Autodesk Inventor part; units mm, degrees
(part 14 of 16)
  arc A294 (20.5053, 59.1049) -> (19.7702, 59.9479) centre (0.0409, 42.0024) ccw
  spline S90 degree 3 poles (17.578, 62.0957) (17.5149, 61.9054) (17.4259, 61.6609) (17.3048, 61.369) (17.2372, 61.2153) (17.171, 61.0728) (17.1066, 60.9415) (17.0444, 60.8212) (16.9848, 60.7117) (16.9284, 60.6129) (16.8755, 60.5246) (16.8265, 60.4466) (16.7818, 60.3788) (16.7419, 60.3207) (16.7071, 60.2724) (16.6673, 60.2192) (16.6296, 60.1737) (16.5954, 60.1304) (16.5731, 60.101) (16.5518, 60.0719) (16.5315, 60.0431) (16.5122, 60.0145) (16.494, 59.9861) (16.4767, 59.9579) (16.4604, 59.9297) (16.4451, 59.9016) (16.4307, 59.8733) (16.4173, 59.8448) (16.4048, 59.8159) (16.3933, 59.7865) (16.3828, 59.7562) (16.3735, 59.7248) (16.3654, 59.6921) (16.3588, 59.6574) (16.354, 59.6205) (16.3517, 59.5807) (16.3525, 59.5377) (16.3576, 59.4911) (16.3684, 59.4408) (16.3865, 59.3878) (16.4133, 59.3335) (16.4479, 59.2826) (16.5472, 59.1764) (16.7178, 59.0249) (16.8727, 58.8575) (16.981, 58.7604) (17.0325, 58.7268) (17.0873, 58.7011) (17.1408, 58.6842) (17.1912, 58.6744) (17.2379, 58.6703) (17.281, 58.6703) (17.3207, 58.6735) (17.3575, 58.679) (17.392, 58.6863) (17.4246, 58.695) (17.4558, 58.705) (17.4858, 58.7161) (17.515, 58.7283) (17.5436, 58.7413) (17.5718, 58.7554) (17.5998, 58.7703) (17.6277, 58.7862) (17.6555, 58.8031) (17.6834, 58.8209) (17.7114, 58.8398) (17.7396, 58.8596) (17.7679, 58.8804) (17.7966, 58.9023) (17.8255, 58.9253) (17.8681, 58.9603) (17.9128, 58.999) (17.9652, 59.0398) (18.0128, 59.0757) (18.07, 59.1168) (18.137, 59.1628) (18.2139, 59.2134) (18.3011, 59.2681) (18.3987, 59.3265) (18.5069, 59.3883) (18.626, 59.453) (18.7559, 59.5201) (18.897, 59.5892) (19.0493, 59.66) (19.3387, 59.787) (19.5813, 59.881) (19.7702, 59.9479) knots 0 0 0 0 0.085622 0.111078 0.134991 0.157361 0.178189 0.197474 0.215216 0.231415 0.246072 0.259186 0.270757 0.280785 0.28927 0.296213 0.309142 0.314525 0.319779 0.32491 0.329923 0.334826 0.339627 0.344336 0.348964 0.353525 0.358035 0.362514 0.366985 0.371475 0.37602 0.380661 0.385447 0.39044 0.395711 0.401345 0.407436 0.41408 0.421363 0.429333 0.437971 0.447155 0.455484 0.5 0.544516 0.552845 0.562029 0.570667 0.578637 0.58592 0.592564 0.598655 0.604289 0.60956 0.614553 0.619339 0.62398 0.628525 0.633015 0.637486 0.641965 0.646475 0.651036 0.655664 0.660373 0.665174 0.670077 0.67509 0.680221 0.685475 0.690858 0.703787 0.71073 0.719215 0.729243 0.740814 0.753928 0.768585 0.784784 0.802526 0.821811 0.842639 0.865009 0.888922 0.914378 1 1 1 1
  arc A295 (17.578, 62.0957) -> (16.72, 62.8133) centre (0.0409, 42.0024) ccw
  spline S91 degree 3 poles (14.2188, 64.5917) (14.1862, 64.3939) (14.1366, 64.1385) (14.0627, 63.8313) (14.02, 63.6688) (13.9768, 63.5178) (13.9337, 63.378) (13.8911, 63.2494) (13.8494, 63.132) (13.8092, 63.0256) (13.7707, 62.9301) (13.7345, 62.8454) (13.701, 62.7714) (13.6707, 62.7078) (13.6439, 62.6546) (13.6129, 62.5959) (13.5828, 62.545) (13.5558, 62.4969) (13.5383, 62.4644) (13.5218, 62.4323) (13.5063, 62.4007) (13.4917, 62.3695) (13.4782, 62.3386) (13.4655, 62.308) (13.4538, 62.2776) (13.4431, 62.2474) (13.4333, 62.2172) (13.4245, 62.187) (13.4167, 62.1565) (13.4099, 62.1256) (13.4043, 62.0941) (13.4, 62.0616) (13.3971, 62.028) (13.396, 61.9927) (13.3971, 61.9555) (13.401, 61.9159) (13.4086, 61.8735) (13.4209, 61.8282) (13.4394, 61.7803) (13.4656, 61.7307) (13.5005, 61.6813) (13.5427, 61.6365) (13.6573, 61.5471) (13.8495, 61.4242) (14.0287, 61.283) (14.1509, 61.2041) (14.207, 61.179) (14.2652, 61.1622) (14.3206, 61.1538) (14.372, 61.152) (14.4188, 61.1553) (14.4613, 61.162) (14.5, 61.1714) (14.5355, 61.1826) (14.5684, 61.1952) (14.5993, 61.2089) (14.6285, 61.2237) (14.6564, 61.2394) (14.6834, 61.2559) (14.7096, 61.2733) (14.7353, 61.2915) (14.7606, 61.3107) (14.7856, 61.3308) (14.8104, 61.3518) (14.8352, 61.3738) (14.8599, 61.3967) (14.8846, 61.4207) (14.9094, 61.4458) (14.9342, 61.4719) (14.9592, 61.499) (14.9958, 61.5404) (15.0339, 61.5855) (15.0792, 61.6341) (15.1207, 61.6769) (15.1708, 61.7264) (15.2297, 61.7824) (15.2978, 61.8444) (15.3753, 61.9121) (15.4626, 61.9851) (15.5598, 62.063) (15.6673, 62.1455) (15.7851, 62.2321) (15.9137, 62.3224) (16.0531, 62.4161) (16.319, 62.5869) (16.5439, 62.7176) (16.72, 62.8133) knots 0 0 0 0 0.085622 0.111078 0.134991 0.157361 0.178189 0.197474 0.215216 0.231415 0.246072 0.259186 0.270757 0.280785 0.28927 0.296213 0.309142 0.314525 0.319779 0.32491 0.329923 0.334826 0.339627 0.344336 0.348964 0.353525 0.358035 0.362514 0.366985 0.371475 0.37602 0.380661 0.385447 0.39044 0.395711 0.401345 0.407436 0.41408 0.421363 0.429333 0.437971 0.447155 0.455484 0.5 0.544516 0.552845 0.562029 0.570667 0.578637 0.58592 0.592564 0.598655 0.604289 0.60956 0.614553 0.619339 0.62398 0.628525 0.633015 0.637486 0.641965 0.646475 0.651036 0.655664 0.660373 0.665174 0.670077 0.67509 0.680221 0.685475 0.690858 0.703787 0.71073 0.719215 0.729243 0.740814 0.753928 0.768585 0.784784 0.802526 0.821811 0.842639 0.865009 0.888922 0.914378 1 1 1 1
  arc A296 (14.2188, 64.5917) -> (13.2591, 65.1663) centre (0.0409, 42.0024) ccw
  spline S92 degree 3 poles (10.5105, 66.5315) (10.5093, 66.331) (10.5002, 66.071) (10.4753, 65.756) (10.4585, 65.5889) (10.4395, 65.4329) (10.4188, 65.2881) (10.3968, 65.1545) (10.374, 65.032) (10.3509, 64.9206) (10.3279, 64.8203) (10.3054, 64.731) (10.2839, 64.6526) (10.2638, 64.5851) (10.2457, 64.5283) (10.2243, 64.4655) (10.2025, 64.4105) (10.1833, 64.3588) (10.1711, 64.3239) (10.1599, 64.2897) (10.1495, 64.256) (10.14, 64.2229) (10.1314, 64.1902) (10.1238, 64.1581) (10.117, 64.1262) (10.1111, 64.0947) (10.1061, 64.0634) (10.1022, 64.0321) (10.0992, 64.0008) (10.0974, 63.9692) (10.0968, 63.9372) (10.0975, 63.9045) (10.1, 63.8708) (10.1044, 63.8358) (10.1113, 63.7992) (10.1213, 63.7607) (10.1354, 63.72) (10.1547, 63.6772) (10.1805, 63.6328) (10.2141, 63.5879) (10.2564, 63.5446) (10.305, 63.5069) (10.4322, 63.4365) (10.6413, 63.3452) (10.8404, 63.2338) (10.9733, 63.175) (11.0327, 63.159) (11.0928, 63.1515) (11.1489, 63.1519) (11.1998, 63.1582) (11.2456, 63.1686) (11.2865, 63.182) (11.3233, 63.1973) (11.3566, 63.2139) (11.3872, 63.2315) (11.4155, 63.2499) (11.442, 63.269) (11.4671, 63.2889) (11.4912, 63.3094) (11.5144, 63.3307) (11.5369, 63.3528) (11.5589, 63.3756) (11.5804, 63.3994) (11.6017, 63.424) (11.6227, 63.4496) (11.6435, 63.4761) (11.6642, 63.5037) (11.6847, 63.5323) (11.7052, 63.562) (11.7256, 63.5927) (11.7553, 63.6393) (11.7859, 63.6899) (11.823, 63.7449) (11.8573, 63.7937) (11.899, 63.8504) (11.9484, 63.9149) (12.006, 63.9868) (12.072, 64.0658) (12.1468, 64.1515) (12.2306, 64.2437) (12.3238, 64.342) (12.4267, 64.446) (12.5395, 64.5553) (12.6625, 64.6697) (12.8984, 64.8799) (13.1001, 65.0442) (13.2591, 65.1663) knots 0 0 0 0 0.085622 0.111078 0.134991 0.157361 0.178189 0.197474 0.215216 0.231415 0.246072 0.259186 0.270757 0.280785 0.28927 0.296213 0.309142 0.314525 0.319779 0.32491 0.329923 0.334826 0.339627 0.344336 0.348964 0.353525 0.358035 0.362514 0.366985 0.371475 0.37602 0.380661 0.385447 0.39044 0.395711 0.401345 0.407436 0.41408 0.421363 0.429333 0.437971 0.447155 0.455484 0.5 0.544516 0.552845 0.562029 0.570667 0.578637 0.58592 0.592564 0.598655 0.604289 0.60956 0.614553 0.619339 0.62398 0.628525 0.633015 0.637486 0.641965 0.646475 0.651036 0.655664 0.660373 0.665174 0.670077 0.67509 0.680221 0.685475 0.690858 0.703787 0.71073 0.719215 0.729243 0.740814 0.753928 0.768585 0.784784 0.802526 0.821811 0.842639 0.865009 0.888922 0.914378 1 1 1 1
  arc A297 (10.5105, 66.5315) -> (9.4727, 66.9489) centre (0.0409, 42.0024) ccw
  spline S93 degree 3 poles (6.5444, 67.8673) (6.5745, 67.6691) (6.6063, 67.4109) (6.6309, 67.0958) (6.6405, 66.9282) (6.6461, 66.7712) (6.6483, 66.6249) (6.6475, 66.4895) (6.6442, 66.3649) (6.6388, 66.2513) (6.6317, 66.1486) (6.6235, 66.0568) (6.6145, 65.9761) (6.6053, 65.9063) (6.5962, 65.8474) (6.5849, 65.7819) (6.572, 65.7242) (6.5611, 65.6701) (6.5546, 65.6338) (6.5488, 65.5982) (6.5438, 65.5634) (6.5396, 65.5292) (6.5363, 65.4956) (6.5337, 65.4626) (6.532, 65.4301) (6.5311, 65.398) (6.5311, 65.3663) (6.5321, 65.3348) (6.5341, 65.3034) (6.5372, 65.2719) (6.5416, 65.2402) (6.5475, 65.208) (6.5552, 65.1751) (6.565, 65.1413) (6.5775, 65.1062) (6.5935, 65.0697) (6.6138, 65.0318) (6.6395, 64.9925) (6.6719, 64.9527) (6.7121, 64.9136) (6.7606, 64.8774) (6.8146, 64.8478) (6.9513, 64.7982) (7.172, 64.7407) (7.3861, 64.6618) (7.5266, 64.6245) (7.5878, 64.618) (7.6483, 64.62) (7.7036, 64.6291) (7.753, 64.6433) (7.7965, 64.6609) (7.8348, 64.6804) (7.8688, 64.7013) (7.8991, 64.7229) (7.9265, 64.7451) (7.9516, 64.7677) (7.9748, 64.7907) (7.9965, 64.8143) (8.0171, 64.8383) (8.0366, 64.863) (8.0554, 64.8883) (8.0735, 64.9143) (8.0911, 64.9411) (8.1083, 64.9688) (8.125, 64.9973) (8.1414, 65.0268) (8.1575, 65.0573) (8.1733, 65.0887) (8.1889, 65.1212) (8.2043, 65.1548) (8.2263, 65.2054) (8.2486, 65.2602) (8.2767, 65.3203) (8.3029, 65.3739) (8.3352, 65.4364) (8.3739, 65.5079) (8.4196, 65.5879) (8.4724, 65.6762) (8.5328, 65.7726) (8.6012, 65.8768) (8.6779, 65.9884) (8.7633, 66.1072) (8.8576, 66.2329) (8.9612, 66.365) (9.1613, 66.6096) (9.3348, 66.8035) (9.4727, 66.9489) knots 0 0 0 0 0.085622 0.111078 0.134991 0.157361 0.178189 0.197474 0.215216 0.231415 0.246072 0.259186 0.270757 0.280785 0.28927 0.296213 0.309142 0.314525 0.319779 0.32491 0.329923 0.334826 0.339627 0.344336 0.348964 0.353525 0.358035 0.362514 0.366985 0.371475 0.37602 0.380661 0.385447 0.39044 0.395711 0.401345 0.407436 0.41408 0.421363 0.429333 0.437971 0.447155 0.455484 0.5 0.544516 0.552845 0.562029 0.570667 0.578637 0.58592 0.592564 0.598655 0.604289 0.60956 0.614553 0.619339 0.62398 0.628525 0.633015 0.637486 0.641965 0.646475 0.651036 0.655664 0.660373 0.665174 0.670077 0.67509 0.680221 0.685475 0.690858 0.703787 0.71073 0.719215 0.729243 0.740814 0.753928 0.768585 0.784784 0.802526 0.821811 0.842639 0.865009 0.888922 0.914378 1 1 1 1
  arc A298 (6.5444, 67.8673) -> (5.4541, 68.1172) centre (0.0409, 42.0024) ccw
  spline S94 degree 3 poles (2.4182, 68.5662) (2.4789, 68.3752) (2.5507, 68.1251) (2.6243, 67.8178) (2.66, 67.6537) (2.6901, 67.4995) (2.7152, 67.3554) (2.7356, 67.2215) (2.7518, 67.0979) (2.7642, 66.9849) (2.7733, 66.8823) (2.7795, 66.7904) (2.7832, 66.7093) (2.7851, 66.6388) (2.7853, 66.5793) (2.7844, 66.5129) (2.7806, 66.4539) (2.7784, 66.3987) (2.7776, 66.3618) (2.7775, 66.3258) (2.778, 66.2906) (2.7792, 66.2561) (2.7812, 66.2224) (2.7838, 66.1894) (2.7872, 66.1571) (2.7913, 66.1253) (2.7963, 66.094) (2.8022, 66.063) (2.809, 66.0323) (2.8171, 66.0017) (2.8264, 65.9711) (2.8372, 65.9402) (2.8499, 65.9089) (2.8649, 65.877) (2.8828, 65.8443) (2.9043, 65.8108) (2.9303, 65.7765) (2.9618, 65.7417) (3.0001, 65.7075) (3.0459, 65.6751) (3.0995, 65.647) (3.1574, 65.6262) (3.3001, 65.5986) (3.5272, 65.5763) (3.7509, 65.5319) (3.8956, 65.517) (3.957, 65.5201) (4.0165, 65.5316) (4.0697, 65.5493) (4.1162, 65.571) (4.1565, 65.5951) (4.1913, 65.6205) (4.2215, 65.6464) (4.2481, 65.6725) (4.2717, 65.6986) (4.2929, 65.7249) (4.3122, 65.7513) (4.33, 65.7779) (4.3465, 65.8049) (4.362, 65.8323) (4.3766, 65.8602) (4.3904, 65.8888) (4.4036, 65.918) (4.4162, 65.948) (4.4283, 65.9789) (4.4399, 66.0105) (4.451, 66.0431) (4.4617, 66.0767) (4.472, 66.1112) (4.4819, 66.1468) (4.4958, 66.2002) (4.5092, 66.2578) (4.5276, 66.3216) (4.5451, 66.3786) (4.5672, 66.4454) (4.5943, 66.522) (4.6268, 66.6082) (4.6652, 66.7037) (4.7098, 66.8084) (4.7611, 66.922) (4.8193, 67.0442) (4.885, 67.1749) (4.9585, 67.3138) (5.0402, 67.4605) (5.1996, 67.7334) (5.3407, 67.952) (5.4541, 68.1172) knots 0 0 0 0 0.085622 0.111078 0.134991 0.157361 0.178189 0.197474 0.215216 0.231415 0.246072 0.259186 0.270757 0.280785 0.28927 0.296213 0.309142 0.314525 0.319779 0.32491 0.329923 0.334826 0.339627 0.344336 0.348964 0.353525 0.358035 0.362514 0.366985 0.371475 0.37602 0.380661 0.385447 0.39044 0.395711 0.401345 0.407436 0.41408 0.421363 0.429333 0.437971 0.447155 0.455484 0.5 0.544516 0.552845 0.562029 0.570667 0.578637 0.58592 0.592564 0.598655 0.604289 0.60956 0.614553 0.619339 0.62398 0.628525 0.633015 0.637486 0.641965 0.646475 0.651036 0.655664 0.660373 0.665174 0.670077 0.67509 0.680221 0.685475 0.690858 0.703787 0.71073 0.719215 0.729243 0.740814 0.753928 0.768585 0.784784 0.802526 0.821811 0.842639 0.865009 0.888922 0.914378 1 1 1 1
  arc A299 (2.4182, 68.5662) -> (1.3022, 68.6425) centre (0.0409, 42.0024) ccw
  spline S95 degree 3 poles (-1.7666, 68.6111) (-1.6767, 68.4319) (-1.5667, 68.1961) (-1.4459, 67.9041) (-1.385, 67.7476) (-1.3311, 67.6) (-1.2838, 67.4616) (-1.2427, 67.3325) (-1.2074, 67.213) (-1.1775, 67.1033) (-1.1525, 67.0034) (-1.132, 66.9137) (-1.1155, 66.8341) (-1.1027, 66.7648) (-1.0932, 66.706) (-1.0837, 66.6403) (-1.0782, 66.5814) (-1.0717, 66.5266) (-1.0667, 66.49) (-1.0612, 66.4544) (-1.0552, 66.4197) (-1.0486, 66.3859) (-1.0414, 66.3529) (-1.0337, 66.3207) (-1.0253, 66.2893) (-1.0162, 66.2585) (-1.0064, 66.2284) (-0.9957, 66.1987) (-0.9841, 66.1695) (-0.9714, 66.1405) (-0.9575, 66.1117) (-0.9419, 66.0829) (-0.9245, 66.054) (-0.9046, 66.0249) (-0.8819, 65.9954) (-0.8554, 65.9656) (-0.8244, 65.9358) (-0.7878, 65.9064) (-0.7447, 65.8785) (-0.6943, 65.8538) (-0.637, 65.8343) (-0.5766, 65.8228) (-0.4313, 65.8179) (-0.2035, 65.8315) (0.0244, 65.8226) (0.1696, 65.8305) (0.2298, 65.8432) (0.2867, 65.8638) (0.3365, 65.8896) (0.3791, 65.9184) (0.4151, 65.9485) (0.4455, 65.979) (0.4713, 66.0093) (0.4935, 66.0392) (0.5127, 66.0687) (0.5295, 66.098) (0.5445, 66.1271) (0.5579, 66.1562) (0.57, 66.1854) (0.581, 66.2149) (0.591, 66.2448) (0.6002, 66.2751) (0.6087, 66.3061) (0.6164, 66.3377) (0.6235, 66.37) (0.63, 66.4031) (0.6359, 66.4371) (0.6412, 66.4719) (0.646, 66.5076) (0.6502, 66.5443) (0.6555, 66.5992) (0.6598, 66.6582) (0.668, 66.7241) (0.6763, 66.7831) (0.6877, 66.8526) (0.7025, 66.9325) (0.7212, 67.0227) (0.7441, 67.123) (0.7718, 67.2334) (0.8047, 67.3535) (0.8431, 67.4834) (0.8876, 67.6228) (0.9384, 67.7714) (0.9961, 67.9292) (1.1109, 68.2236) (1.216, 68.4616) (1.3022, 68.6425) knots 0 0 0 0 0.085622 0.111078 0.134991 0.157361 0.178189 0.197474 0.215216 0.231415 0.246072 0.259186 0.270757 0.280785 0.28927 0.296213 0.309142 0.314525 0.319779 0.32491 0.329923 0.334826 0.339627 0.344336 0.348964 0.353525 0.358035 0.362514 0.366985 0.371475 0.37602 0.380661 0.385447 0.39044 0.395711 0.401345 0.407436 0.41408 0.421363 0.429333 0.437971 0.447155 0.455484 0.5 0.544516 0.552845 0.562029 0.570667 0.578637 0.58592 0.592564 0.598655 0.604289 0.60956 0.614553 0.619339 0.62398 0.628525 0.633015 0.637486 0.641965 0.646475 0.651036 0.655664 0.660373 0.665174 0.670077 0.67509 0.680221 0.685475 0.690858 0.703787 0.71073 0.719215 0.729243 0.740814 0.753928 0.768585 0.784784 0.802526 0.821811 0.842639 0.865009 0.888922 0.914378 1 1 1 1
  arc A300 (-1.7666, 68.6111) -> (-2.8808, 68.5119) centre (0.0409, 42.0024) ccw
  spline S96 degree 3 poles (-5.9069, 68.0007) (-5.79, 67.8378) (-5.6445, 67.6222) (-5.4796, 67.3526) (-5.3949, 67.2076) (-5.3186, 67.0702) (-5.2502, 66.9409) (-5.1894, 66.8199) (-5.1359, 66.7074) (-5.0891, 66.6037) (-5.0488, 66.509) (-5.0145, 66.4235) (-4.9858, 66.3474) (-4.9623, 66.281) (-4.9437, 66.2244) (-4.924, 66.161) (-4.9094, 66.1037) (-4.8945, 66.0506) (-4.8838, 66.0153) (-4.8728, 65.9809) (-4.8614, 65.9476) (-4.8496, 65.9153) (-4.8374, 65.8838) (-4.8247, 65.8532) (-4.8115, 65.8235) (-4.7977, 65.7945) (-4.7833, 65.7663) (-4.7681, 65.7387) (-4.7521, 65.7116) (-4.735, 65.685) (-4.7167, 65.6587) (-4.6968, 65.6327) (-4.6751, 65.6069) (-4.6509, 65.5812) (-4.6238, 65.5556) (-4.5931, 65.5304) (-4.5577, 65.5057) (-4.517, 65.4825) (-4.47, 65.4617) (-4.4165, 65.4451) (-4.3568, 65.4349) (-4.2953, 65.433) (-4.151, 65.4508) (-3.9282, 65.4998) (-3.7017, 65.5267) (-3.5595, 65.5573) (-3.5021, 65.5792) (-3.449, 65.6085) (-3.4039, 65.6418) (-3.3664, 65.6768) (-3.3355, 65.7122) (-3.3103, 65.7471) (-3.2895, 65.781) (-3.2723, 65.8141) (-3.2579, 65.8463) (-3.2459, 65.8778) (-3.2356, 65.9089) (-3.227, 65.9397) (-3.2196, 65.9704) (-3.2133, 66.0013) (-3.2081, 66.0324) (-3.2038, 66.0638) (-3.2003, 66.0957) (-3.1976, 66.1281) (-3.1956, 66.1611) (-3.1944, 66.1948) (-3.1938, 66.2293) (-3.194, 66.2645) (-3.1949, 66.3006) (-3.1965, 66.3374) (-3.1998, 66.3925) (-3.2048, 66.4514) (-3.2071, 66.5178) (-3.208, 66.5774) (-3.2077, 66.6478) (-3.2056, 66.729) (-3.2012, 66.821) (-3.1943, 66.9237) (-3.1842, 67.0371) (-3.1705, 67.1609) (-3.1529, 67.2952) (-3.1308, 67.4398) (-3.1038, 67.5946) (-3.0715, 67.7594) (-3.0042, 68.0682) (-2.9376, 68.3197) (-2.8808, 68.5119) knots 0 0 0 0 0.085622 0.111078 0.134991 0.157361 0.178189 0.197474 0.215216 0.231415 0.246072 0.259186 0.270757 0.280785 0.28927 0.296213 0.309142 0.314525 0.319779 0.32491 0.329923 0.334826 0.339627 0.344336 0.348964 0.353525 0.358035 0.362514 0.366985 0.371475 0.37602 0.380661 0.385447 0.39044 0.395711 0.401345 0.407436 0.41408 0.421363 0.429333 0.437971 0.447155 0.455484 0.5 0.544516 0.552845 0.562029 0.570667 0.578637 0.58592 0.592564 0.598655 0.604289 0.60956 0.614553 0.619339 0.62398 0.628525 0.633015 0.637486 0.641965 0.646475 0.651036 0.655664 0.660373 0.665174 0.670077 0.67509 0.680221 0.685475 0.690858 0.703787 0.71073 0.719215 0.729243 0.740814 0.753928 0.768585 0.784784 0.802526 0.821811 0.842639 0.865009 0.888922 0.914378 1 1 1 1
  arc A301 (-5.9069, 68.0007) -> (-6.9918, 67.7284) centre (0.0409, 42.0024) ccw
  spline S97 degree 3 poles (-9.9007, 66.7502) (-9.7598, 66.6076) (-9.5823, 66.4173) (-9.3772, 66.1769) (-9.2709, 66.0469) (-9.1741, 65.9232) (-9.0863, 65.8062) (-9.0074, 65.6961) (-8.9368, 65.5934) (-8.8744, 65.4983) (-8.8198, 65.411) (-8.7726, 65.332) (-8.7323, 65.2614) (-8.6987, 65.1995) (-8.6715, 65.1465) (-8.6421, 65.0869) (-8.6187, 65.0326) (-8.5957, 64.9825) (-8.5796, 64.9492) (-8.5634, 64.9171) (-8.5469, 64.8859) (-8.5302, 64.8558) (-8.5132, 64.8267) (-8.4959, 64.7985) (-8.4782, 64.7712) (-8.46, 64.7447) (-8.4414, 64.719) (-8.4221, 64.6941) (-8.402, 64.6699) (-8.381, 64.6463) (-8.3588, 64.6232) (-8.3351, 64.6006) (-8.3096, 64.5785) (-8.2817, 64.5569) (-8.251, 64.5359) (-8.2166, 64.5158) (-8.1779, 64.497) (-8.134, 64.4804) (-8.0843, 64.4672) (-8.0288, 64.4592) (-7.9683, 64.4584) (-7.9073, 64.4662) (-7.7676, 64.5064) (-7.5552, 64.5896) (-7.3356, 64.6516) (-7.2, 64.704) (-7.1467, 64.7347) (-7.0989, 64.7719) (-7.0595, 64.8118) (-7.0279, 64.8523) (-7.003, 64.8921) (-6.9835, 64.9305) (-6.9683, 64.9673) (-6.9565, 65.0026) (-6.9473, 65.0366) (-6.9403, 65.0697) (-6.9351, 65.102) (-6.9313, 65.1338) (-6.9289, 65.1653) (-6.9275, 65.1967) (-6.9272, 65.2283) (-6.9278, 65.26) (-6.9294, 65.292) (-6.9318, 65.3245) (-6.935, 65.3574) (-6.9391, 65.3909) (-6.9439, 65.425) (-6.9496, 65.4598) (-6.9561, 65.4952) (-6.9635, 65.5314) (-6.9754, 65.5853) (-6.9895, 65.6427) (-7.0021, 65.7079) (-7.0124, 65.7666) (-7.0231, 65.8362) (-7.0337, 65.9168) (-7.0438, 66.0083) (-7.053, 66.1108) (-7.0608, 66.2243) (-7.0667, 66.3488) (-7.0702, 66.4842) (-7.071, 66.6305) (-7.0686, 66.7875) (-7.0625, 66.9554) (-7.0443, 67.2709) (-7.0179, 67.5297) (-6.9918, 67.7284) knots 0 0 0 0 0.085622 0.111078 0.134991 0.157361 0.178189 0.197474 0.215216 0.231415 0.246072 0.259186 0.270757 0.280785 0.28927 0.296213 0.309142 0.314525 0.319779 0.32491 0.329923 0.334826 0.339627 0.344336 0.348964 0.353525 0.358035 0.362514 0.366985 0.371475 0.37602 0.380661 0.385447 0.39044 0.395711 0.401345 0.407436 0.41408 0.421363 0.429333 0.437971 0.447155 0.455484 0.5 0.544516 0.552845 0.562029 0.570667 0.578637 0.58592 0.592564 0.598655 0.604289 0.60956 0.614553 0.619339 0.62398 0.628525 0.633015 0.637486 0.641965 0.646475 0.651036 0.655664 0.660373 0.665174 0.670077 0.67509 0.680221 0.685475 0.690858 0.703787 0.71073 0.719215 0.729243 0.740814 0.753928 0.768585 0.784784 0.802526 0.821811 0.842639 0.865009 0.888922 0.914378 1 1 1 1
  arc A302 (-9.9007, 66.7502) -> (-10.9296, 66.3116) centre (0.0409, 42.0024) ccw
  spline S98 degree 3 poles (-13.6497, 64.8903) (-13.4883, 64.7715) (-13.2832, 64.6113) (-13.043, 64.406) (-12.9177, 64.2942) (-12.8027, 64.1872) (-12.6977, 64.0853) (-12.6025, 63.989) (-12.5168, 63.8985) (-12.4402, 63.8143) (-12.3726, 63.7367) (-12.3136, 63.666) (-12.2628, 63.6026) (-12.22, 63.5467) (-12.1847, 63.4986) (-12.1465, 63.4444) (-12.1148, 63.3944) (-12.0842, 63.3485) (-12.0632, 63.3182) (-12.0421, 63.2889) (-12.021, 63.2608) (-11.9997, 63.2336) (-11.9784, 63.2075) (-11.9569, 63.1824) (-11.9351, 63.1582) (-11.913, 63.1349) (-11.8906, 63.1124) (-11.8677, 63.0909) (-11.844, 63.0701) (-11.8196, 63.05) (-11.794, 63.0307) (-11.7671, 63.0121) (-11.7384, 62.9943) (-11.7076, 62.9773) (-11.6739, 62.9614) (-11.6368, 62.9468) (-11.5956, 62.9343) (-11.5497, 62.9248) (-11.4986, 62.9195) (-11.4425, 62.9203) (-11.3826, 62.929) (-11.3235, 62.9462) (-11.1918, 63.0078) (-10.9951, 63.1233) (-10.7879, 63.2189) (-10.6621, 63.2918) (-10.6143, 63.3305) (-10.5729, 63.3747) (-10.5403, 63.4203) (-10.5154, 63.4652) (-10.497, 63.5084) (-10.4837, 63.5493) (-10.4745, 63.5881) (-10.4683, 63.6248) (-10.4646, 63.6599) (-10.4629, 63.6936) (-10.4628, 63.7263) (-10.4641, 63.7583) (-10.4665, 63.7898) (-10.4701, 63.8211) (-10.4748, 63.8523) (-10.4803, 63.8835) (-10.4869, 63.9149) (-10.4943, 63.9466) (-10.5027, 63.9786) (-10.5119, 64.011) (-10.5221, 64.044) (-10.5331, 64.0774) (-10.5451, 64.1114) (-10.558, 64.146) (-10.5782, 64.1973) (-10.6011, 64.2518) (-10.6238, 64.3142) (-10.6431, 64.3706) (-10.6645, 64.4377) (-10.6876, 64.5156) (-10.7119, 64.6044) (-10.737, 64.7043) (-10.7625, 64.8152) (-10.7878, 64.9372) (-10.8125, 65.0703) (-10.8361, 65.2147) (-10.8583, 65.3702) (-10.8785, 65.537) (-10.9099, 65.8514) (-10.9243, 66.1112) (-10.9296, 66.3116) knots 0 0 0 0 0.085622 0.111078 0.134991 0.157361 0.178189 0.197474 0.215216 0.231415 0.246072 0.259186 0.270757 0.280785 0.28927 0.296213 0.309142 0.314525 0.319779 0.32491 0.329923 0.334826 0.339627 0.344336 0.348964 0.353525 0.358035 0.362514 0.366985 0.371475 0.37602 0.380661 0.385447 0.39044 0.395711 0.401345 0.407436 0.41408 0.421363 0.429333 0.437971 0.447155 0.455484 0.5 0.544516 0.552845 0.562029 0.570667 0.578637 0.58592 0.592564 0.598655 0.604289 0.60956 0.614553 0.619339 0.62398 0.628525 0.633015 0.637486 0.641965 0.646475 0.651036 0.655664 0.660373 0.665174 0.670077 0.67509 0.680221 0.685475 0.690858 0.703787 0.71073 0.719215 0.729243 0.740814 0.753928 0.768585 0.784784 0.802526 0.821811 0.842639 0.865009 0.888922 0.914378 1 1 1 1
  arc A303 (-13.6497, 64.8903) -> (-14.5974, 64.2961) centre (0.0409, 42.0024) ccw
  spline S99 degree 3 poles (-17.0616, 62.4668) (-16.8836, 62.3747) (-16.656, 62.2486) (-16.3866, 62.0834) (-16.2453, 61.9926) (-16.115, 61.9049) (-15.9954, 61.8207) (-15.8863, 61.7404) (-15.7875, 61.6645) (-15.6987, 61.5933) (-15.6198, 61.5272) (-15.5504, 61.4666) (-15.4904, 61.4119) (-15.4393, 61.3634) (-15.397, 61.3214) (-15.3507, 61.2739) (-15.3116, 61.2295) (-15.2742, 61.1889) (-15.2487, 61.1622) (-15.2233, 61.1367) (-15.198, 61.1121) (-15.1728, 61.0887) (-15.1476, 61.0662) (-15.1224, 61.0447) (-15.0971, 61.0242) (-15.0717, 61.0047) (-15.046, 60.986) (-15.02, 60.9683) (-14.9934, 60.9515) (-14.9661, 60.9355) (-14.9379, 60.9204) (-14.9084, 60.9063) (-14.8773, 60.8931) (-14.8441, 60.8812) (-14.8084, 60.8707) (-14.7695, 60.8622) (-14.7268, 60.8563) (-14.6799, 60.854) (-14.6287, 60.8568) (-14.5734, 60.8664) (-14.5156, 60.8844) (-14.46, 60.9106) (-14.3395, 60.992) (-14.1632, 61.1368) (-13.9736, 61.2636) (-13.8608, 61.3554) (-13.8196, 61.4011) (-13.7856, 61.4512) (-13.7605, 61.5013) (-13.743, 61.5496) (-13.7315, 61.5951) (-13.7249, 61.6376) (-13.7218, 61.6773) (-13.7214, 61.7146) (-13.7233, 61.7498) (-13.7268, 61.7834) (-13.7318, 61.8157) (-13.7381, 61.8471) (-13.7455, 61.8778) (-13.7539, 61.9082) (-13.7634, 61.9382) (-13.7738, 61.9682) (-13.7851, 61.9982) (-13.7974, 62.0283) (-13.8107, 62.0586) (-13.8249, 62.0892) (-13.8401, 62.1202) (-13.8562, 62.1515) (-13.8734, 62.1832) (-13.8915, 62.2153) (-13.9195, 62.2629) (-13.9507, 62.3131) (-13.9828, 62.3712) (-14.0107, 62.4239) (-14.0424, 62.4868) (-14.0774, 62.5601) (-14.1153, 62.6441) (-14.1557, 62.7387) (-14.1982, 62.8443) (-14.2422, 62.9608) (-14.2875, 63.0885) (-14.3334, 63.2274) (-14.3797, 63.3775) (-14.4257, 63.539) (-14.5059, 63.8447) (-14.5607, 64.099) (-14.5974, 64.2961) knots 0 0 0 0 0.085622 0.111078 0.134991 0.157361 0.178189 0.197474 0.215216 0.231415 0.246072 0.259186 0.270757 0.280785 0.28927 0.296213 0.309142 0.314525 0.319779 0.32491 0.329923 0.334826 0.339627 0.344336 0.348964 0.353525 0.358035 0.362514 0.366985 0.371475 0.37602 0.380661 0.385447 0.39044 0.395711 0.401345 0.407436 0.41408 0.421363 0.429333 0.437971 0.447155 0.455484 0.5 0.544516 0.552845 0.562029 0.570667 0.578637 0.58592 0.592564 0.598655 0.604289 0.60956 0.614553 0.619339 0.62398 0.628525 0.633015 0.637486 0.641965 0.646475 0.651036 0.655664 0.660373 0.665174 0.670077 0.67509 0.680221 0.685475 0.690858 0.703787 0.71073 0.719215 0.729243 0.740814 0.753928 0.768585 0.784784 0.802526 0.821811 0.842639 0.865009 0.888922 0.914378 1 1 1 1
  arc A304 (-17.0616, 62.4668) -> (-17.9046, 61.7317) centre (0.0409, 42.0024) ccw
  spline S100 degree 3 poles (-20.0524, 59.5395) (-19.8621, 59.4763) (-19.6176, 59.3874) (-19.3257, 59.2663) (-19.172, 59.1987) (-19.0295, 59.1325) (-18.8982, 59.068) (-18.7779, 59.0058) (-18.6684, 58.9463) (-18.5696, 58.8899) (-18.4813, 58.837) (-18.4034, 58.788) (-18.3355, 58.7433) (-18.2774, 58.7034) (-18.2291, 58.6686) (-18.1759, 58.6288) (-18.1304, 58.5911) (-18.0871, 58.5569) (-18.0577, 58.5345) (-18.0286, 58.5132) (-17.9998, 58.493) (-17.9712, 58.4737) (-17.9429, 58.4555) (-17.9146, 58.4382) (-17.8864, 58.4219) (-17.8583, 58.4066) (-17.83, 58.3922) (-17.8015, 58.3788) (-17.7726, 58.3663) (-17.7432, 58.3548) (-17.7129, 58.3443) (-17.6816, 58.3349) (-17.6488, 58.3268) (-17.6141, 58.3202) (-17.5772, 58.3155) (-17.5375, 58.3131) (-17.4944, 58.314) (-17.4478, 58.3191) (-17.3975, 58.3299) (-17.3445, 58.3479) (-17.2902, 58.3748) (-17.2393, 58.4094) (-17.1331, 58.5086) (-16.9816, 58.6792) (-16.8142, 58.8342) (-16.7171, 58.9424) (-16.6835, 58.994) (-16.6578, 59.0488) (-16.6409, 59.1022) (-16.6311, 59.1527) (-16.627, 59.1994) (-16.627, 59.2425) (-16.6302, 59.2822) (-16.6357, 59.319) (-16.643, 59.3535) (-16.6517, 59.3861) (-16.6618, 59.4172) (-16.6728, 59.4473) (-16.685, 59.4765) (-16.698, 59.5051) (-16.7121, 59.5333) (-16.727, 59.5613) (-16.7429, 59.5891) (-16.7598, 59.617) (-16.7776, 59.6449) (-16.7965, 59.6729) (-16.8163, 59.701) (-16.8371, 59.7294) (-16.859, 59.7581) (-16.882, 59.787) (-16.9171, 59.8296) (-16.9557, 59.8743) (-16.9966, 59.9266) (-17.0324, 59.9743) (-17.0735, 60.0315) (-17.1195, 60.0984) (-17.1701, 60.1754) (-17.2248, 60.2626) (-17.2833, 60.3602) (-17.345, 60.4684) (-17.4097, 60.5874) (-17.4768, 60.7174) (-17.5459, 60.8585) (-17.6167, 61.0108) (-17.7437, 61.3002) (-17.8377, 61.5428) (-17.9046, 61.7317) knots 0 0 0 0 0.085622 0.111078 0.134991 0.157361 0.178189 0.197474 0.215216 0.231415 0.246072 0.259186 0.270757 0.280785 0.28927 0.296213 0.309142 0.314525 0.319779 0.32491 0.329923 0.334826 0.339627 0.344336 0.348964 0.353525 0.358035 0.362514 0.366985 0.371475 0.37602 0.380661 0.385447 0.39044 0.395711 0.401345 0.407436 0.41408 0.421363 0.429333 0.437971 0.447155 0.455484 0.5 0.544516 0.552845 0.562029 0.570667 0.578637 0.58592 0.592564 0.598655 0.604289 0.60956 0.614553 0.619339 0.62398 0.628525 0.633015 0.637486 0.641965 0.646475 0.651036 0.655664 0.660373 0.665174 0.670077 0.67509 0.680221 0.685475 0.690858 0.703787 0.71073 0.719215 0.729243 0.740814 0.753928 0.768585 0.784784 0.802526 0.821811 0.842639 0.865009 0.888922 0.914378 1 1 1 1
  arc A305 (-20.0524, 59.5395) -> (-20.7701, 58.6815) centre (0.0409, 42.0024) ccw
  spline S101 degree 3 poles (-22.5484, 56.1803) (-22.3506, 56.1477) (-22.0952, 56.0981) (-21.788, 56.0242) (-21.6255, 55.9814) (-21.4745, 55.9383) (-21.3347, 55.8952) (-21.2061, 55.8526) (-21.0887, 55.8109) (-20.9823, 55.7706) (-20.8868, 55.7322) (-20.8021, 55.696) (-20.7281, 55.6625) (-20.6645, 55.6322) (-20.6113, 55.6053) (-20.5526, 55.5744) (-20.5017, 55.5442) (-20.4536, 55.5172) (-20.4211, 55.4998) (-20.389, 55.4833) (-20.3574, 55.4678) (-20.3262, 55.4532) (-20.2953, 55.4396) (-20.2647, 55.427) (-20.2343, 55.4153) (-20.2041, 55.4046) (-20.1739, 55.3948) (-20.1437, 55.386) (-20.1132, 55.3782) (-20.0823, 55.3714) (-20.0508, 55.3658) (-20.0183, 55.3614) (-19.9847, 55.3586) (-19.9495, 55.3575) (-19.9122, 55.3586) (-19.8726, 55.3625) (-19.8302, 55.37) (-19.7849, 55.3824) (-19.737, 55.4009) (-19.6874, 55.427) (-19.638, 55.462) (-19.5932, 55.5041) (-19.5038, 55.6188) (-19.3809, 55.811) (-19.2397, 55.9902) (-19.1608, 56.1123) (-19.1357, 56.1685) (-19.1189, 56.2267) (-19.1105, 56.2821) (-19.1088, 56.3334) (-19.112, 56.3803) (-19.1187, 56.4228) (-19.1281, 56.4615) (-19.1393, 56.497) (-19.1519, 56.5299) (-19.1656, 56.5608) (-19.1804, 56.59) (-19.1961, 56.6179) (-19.2126, 56.6448) (-19.23, 56.6711) (-19.2482, 56.6967) (-19.2674, 56.722) (-19.2875, 56.7471) (-19.3085, 56.7719) (-19.3305, 56.7966) (-19.3534, 56.8214) (-19.3774, 56.8461) (-19.4025, 56.8709) (-19.4286, 56.8957) (-19.4558, 56.9207) (-19.4971, 56.9573) (-19.5422, 56.9954) (-19.5908, 57.0407) (-19.6336, 57.0822) (-19.6831, 57.1322) (-19.7391, 57.1912) (-19.8011, 57.2593) (-19.8688, 57.3368) (-19.9418, 57.4241) (-20.0197, 57.5213) (-20.1022, 57.6288) (-20.1888, 57.7466) (-20.2791, 57.8752) (-20.3728, 58.0145) (-20.5436, 58.2804) (-20.6743, 58.5054) (-20.7701, 58.6815) knots 0 0 0 0 0.085622 0.111078 0.134991 0.157361 0.178189 0.197474 0.215216 0.231415 0.246072 0.259186 0.270757 0.280785 0.28927 0.296213 0.309142 0.314525 0.319779 0.32491 0.329923 0.334826 0.339627 0.344336 0.348964 0.353525 0.358035 0.362514 0.366985 0.371475 0.37602 0.380661 0.385447 0.39044 0.395711 0.401345 0.407436 0.41408 0.421363 0.429333 0.437971 0.447155 0.455484 0.5 0.544516 0.552845 0.562029 0.570667 0.578637 0.58592 0.592564 0.598655 0.604289 0.60956 0.614553 0.619339 0.62398 0.628525 0.633015 0.637486 0.641965 0.646475 0.651036 0.655664 0.660373 0.665174 0.670077 0.67509 0.680221 0.685475 0.690858 0.703787 0.71073 0.719215 0.729243 0.740814 0.753928 0.768585 0.784784 0.802526 0.821811 0.842639 0.865009 0.888922 0.914378 1 1 1 1
  arc A306 (-22.5484, 56.1803) -> (-23.123, 55.2206) centre (0.0409, 42.0024) ccw
  spline S102 degree 3 poles (-24.4882, 52.472) (-24.2878, 52.4707) (-24.0277, 52.4617) (-23.7127, 52.4367) (-23.5456, 52.42) (-23.3896, 52.401) (-23.2448, 52.3803) (-23.1112, 52.3583) (-22.9887, 52.3355) (-22.8773, 52.3124) (-22.777, 52.2893) (-22.6877, 52.2668) (-22.6093, 52.2453) (-22.5418, 52.2253) (-22.485, 52.2071) (-22.4222, 52.1858) (-22.3672, 52.1639) (-22.3155, 52.1448) (-22.2806, 52.1326) (-22.2464, 52.1213) (-22.2127, 52.111) (-22.1796, 52.1015) (-22.1469, 52.0929) (-22.1148, 52.0852) (-22.0829, 52.0784) (-22.0514, 52.0726) (-22.0201, 52.0676) (-21.9888, 52.0636) (-21.9575, 52.0607) (-21.9259, 52.0588) (-21.8939, 52.0582) (-21.8612, 52.059) (-21.8275, 52.0614) (-21.7925, 52.0659) (-21.7559, 52.0728) (-21.7174, 52.0828) (-21.6767, 52.0969) (-21.6339, 52.1162) (-21.5895, 52.142) (-21.5446, 52.1756) (-21.5013, 52.2178) (-21.4636, 52.2665) (-21.3932, 52.3937) (-21.3019, 52.6028) (-21.1905, 52.8019) (-21.1317, 52.9348) (-21.1157, 52.9942) (-21.1082, 53.0543) (-21.1086, 53.1104) (-21.1149, 53.1613) (-21.1254, 53.2071) (-21.1387, 53.248) (-21.154, 53.2848) (-21.1706, 53.3181) (-21.1882, 53.3486) (-21.2066, 53.3769) (-21.2257, 53.4035) (-21.2456, 53.4286) (-21.2661, 53.4527) (-21.2874, 53.4758) (-21.3095, 53.4983) (-21.3323, 53.5203) (-21.3561, 53.5419) (-21.3807, 53.5631) (-21.4063, 53.5842) (-21.4329, 53.605) (-21.4604, 53.6256) (-21.489, 53.6462) (-21.5187, 53.6667) (-21.5495, 53.6871) (-21.596, 53.7167) (-21.6466, 53.7473) (-21.7016, 53.7845) (-21.7504, 53.8187) (-21.8071, 53.8604) (-21.8716, 53.9099) (-21.9435, 53.9675) (-22.0225, 54.0335) (-22.1082, 54.1082) (-22.2004, 54.1921) (-22.2987, 54.2853) (-22.4027, 54.3882) (-22.512, 54.501) (-22.6264, 54.624) (-22.8366, 54.8599) (-23.0009, 55.0616) (-23.123, 55.2206) knots 0 0 0 0 0.085622 0.111078 0.134991 0.157361 0.178189 0.197474 0.215216 0.231415 0.246072 0.259186 0.270757 0.280785 0.28927 0.296213 0.309142 0.314525 0.319779 0.32491 0.329923 0.334826 0.339627 0.344336 0.348964 0.353525 0.358035 0.362514 0.366985 0.371475 0.37602 0.380661 0.385447 0.39044 0.395711 0.401345 0.407436 0.41408 0.421363 0.429333 0.437971 0.447155 0.455484 0.5 0.544516 0.552845 0.562029 0.570667 0.578637 0.58592 0.592564 0.598655 0.604289 0.60956 0.614553 0.619339 0.62398 0.628525 0.633015 0.637486 0.641965 0.646475 0.651036 0.655664 0.660373 0.665174 0.670077 0.67509 0.680221 0.685475 0.690858 0.703787 0.71073 0.719215 0.729243 0.740814 0.753928 0.768585 0.784784 0.802526 0.821811 0.842639 0.865009 0.888922 0.914378 1 1 1 1
  arc A307 (-24.4882, 52.472) -> (-24.9056, 51.4342) centre (0.0409, 42.0024) ccw
  spline S103 degree 3 poles (-25.824, 48.5059) (-25.6258, 48.536) (-25.3676, 48.5678) (-25.0526, 48.5924) (-24.8849, 48.602) (-24.7279, 48.6076) (-24.5816, 48.6098) (-24.4462, 48.609) (-24.3216, 48.6057) (-24.208, 48.6002) (-24.1053, 48.5932) (-24.0135, 48.5849) (-23.9328, 48.576) (-23.863, 48.5667) (-23.8041, 48.5577) (-23.7386, 48.5464) (-23.6809, 48.5334) (-23.6268, 48.5226) (-23.5905, 48.516) (-23.5549, 48.5103) (-23.5201, 48.5053) (-23.4859, 48.5011) (-23.4523, 48.4977) (-23.4193, 48.4952) (-23.3868, 48.4935) (-23.3547, 48.4926) (-23.323, 48.4926) (-23.2915, 48.4936) (-23.2601, 48.4956) (-23.2286, 48.4987) (-23.1969, 48.5031) (-23.1647, 48.509) (-23.1319, 48.5166) (-23.098, 48.5265) (-23.0629, 48.539) (-23.0265, 48.555) (-22.9885, 48.5753) (-22.9492, 48.601) (-22.9094, 48.6334) (-22.8703, 48.6736) (-22.8341, 48.7221) (-22.8045, 48.776) (-22.7549, 48.9127) (-22.6974, 49.1335) (-22.6185, 49.3476) (-22.5812, 49.4881) (-22.5747, 49.5493) (-22.5767, 49.6098) (-22.5858, 49.6651) (-22.6, 49.7144) (-22.6176, 49.758) (-22.6371, 49.7963) (-22.658, 49.8303) (-22.6796, 49.8606) (-22.7018, 49.888) (-22.7244, 49.9131) (-22.7474, 49.9363) (-22.771, 49.958) (-22.795, 49.9785) (-22.8197, 49.9981) (-22.845, 50.0169) (-22.871, 50.035) (-22.8978, 50.0526) (-22.9255, 50.0697) (-22.954, 50.0865) (-22.9835, 50.1029) (-23.014, 50.119) (-23.0454, 50.1348) (-23.078, 50.1504) (-23.1115, 50.1657) (-23.1621, 50.1878) (-23.2169, 50.2101) (-23.277, 50.2382) (-23.3306, 50.2644) (-23.3931, 50.2967) (-23.4646, 50.3354) (-23.5446, 50.381) (-23.6329, 50.4339) (-23.7293, 50.4943) (-23.8335, 50.5627) (-23.9451, 50.6394) (-24.0639, 50.7247) (-24.1896, 50.819) (-24.3217, 50.9226) (-24.5663, 51.1228) (-24.7602, 51.2963) (-24.9056, 51.4342) knots 0 0 0 0 0.085622 0.111078 0.134991 0.157361 0.178189 0.197474 0.215216 0.231415 0.246072 0.259186 0.270757 0.280785 0.28927 0.296213 0.309142 0.314525 0.319779 0.32491 0.329923 0.334826 0.339627 0.344336 0.348964 0.353525 0.358035 0.362514 0.366985 0.371475 0.37602 0.380661 0.385447 0.39044 0.395711 0.401345 0.407436 0.41408 0.421363 0.429333 0.437971 0.447155 0.455484 0.5 0.544516 0.552845 0.562029 0.570667 0.578637 0.58592 0.592564 0.598655 0.604289 0.60956 0.614553 0.619339 0.62398 0.628525 0.633015 0.637486 0.641965 0.646475 0.651036 0.655664 0.660373 0.665174 0.670077 0.67509 0.680221 0.685475 0.690858 0.703787 0.71073 0.719215 0.729243 0.740814 0.753928 0.768585 0.784784 0.802526 0.821811 0.842639 0.865009 0.888922 0.914378 1 1 1 1
  arc A308 (-25.824, 48.5059) -> (-26.074, 47.4156) centre (0.0409, 42.0024) ccw
  spline S104 degree 3 poles (-26.5229, 44.3796) (-26.3319, 44.4404) (-26.0818, 44.5122) (-25.7745, 44.5858) (-25.6104, 44.6214) (-25.4562, 44.6516) (-25.3121, 44.6767) (-25.1782, 44.6971) (-25.0547, 44.7132) (-24.9416, 44.7257) (-24.839, 44.7347) (-24.7471, 44.7409) (-24.666, 44.7447) (-24.5956, 44.7465) (-24.536, 44.7468) (-24.4696, 44.7459) (-24.4106, 44.7421) (-24.3554, 44.7399) (-24.3185, 44.7391) (-24.2825, 44.7389) (-24.2473, 44.7395) (-24.2128, 44.7407) (-24.1791, 44.7426) (-24.1462, 44.7453) (-24.1138, 44.7486) (-24.082, 44.7528) (-24.0507, 44.7578) (-24.0197, 44.7637) (-23.989, 44.7705) (-23.9584, 44.7785) (-23.9278, 44.7878) (-23.8969, 44.7987) (-23.8656, 44.8114) (-23.8337, 44.8264) (-23.801, 44.8443) (-23.7675, 44.8658) (-23.7332, 44.8917) (-23.6984, 44.9233) (-23.6642, 44.9615) (-23.6318, 45.0074) (-23.6037, 45.061) (-23.5829, 45.1188) (-23.5553, 45.2616) (-23.533, 45.4887) (-23.4886, 45.7124) (-23.4737, 45.8571) (-23.4769, 45.9185) (-23.4883, 45.9779) (-23.506, 46.0311) (-23.5277, 46.0777) (-23.5518, 46.1179) (-23.5772, 46.1527) (-23.6031, 46.183) (-23.6292, 46.2096) (-23.6554, 46.2332) (-23.6816, 46.2544) (-23.708, 46.2737) (-23.7347, 46.2915) (-23.7616, 46.308) (-23.789, 46.3235) (-23.817, 46.3381) (-23.8455, 46.3519) (-23.8747, 46.3651) (-23.9047, 46.3777) (-23.9356, 46.3898) (-23.9672, 46.4013) (-23.9998, 46.4125) (-24.0334, 46.4232) (-24.068, 46.4335) (-24.1035, 46.4434) (-24.1569, 46.4572) (-24.2145, 46.4707) (-24.2783, 46.4891) (-24.3353, 46.5065) (-24.4021, 46.5287) (-24.4787, 46.5558) (-24.5649, 46.5883) (-24.6604, 46.6267) (-24.7651, 46.6713) (-24.8787, 46.7225) (-25.0009, 46.7808) (-25.1316, 46.8465) (-25.2705, 46.92) (-25.4172, 47.0017) (-25.6901, 47.1611) (-25.9087, 47.3021) (-26.074, 47.4156) knots 0 0 0 0 0.085622 0.111078 0.134991 0.157361 0.178189 0.197474 0.215216 0.231415 0.246072 0.259186 0.270757 0.280785 0.28927 0.296213 0.309142 0.314525 0.319779 0.32491 0.329923 0.334826 0.339627 0.344336 0.348964 0.353525 0.358035 0.362514 0.366985 0.371475 0.37602 0.380661 0.385447 0.39044 0.395711 0.401345 0.407436 0.41408 0.421363 0.429333 0.437971 0.447155 0.455484 0.5 0.544516 0.552845 0.562029 0.570667 0.578637 0.58592 0.592564 0.598655 0.604289 0.60956 0.614553 0.619339 0.62398 0.628525 0.633015 0.637486 0.641965 0.646475 0.651036 0.655664 0.660373 0.665174 0.670077 0.67509 0.680221 0.685475 0.690858 0.703787 0.71073 0.719215 0.729243 0.740814 0.753928 0.768585 0.784784 0.802526 0.821811 0.842639 0.865009 0.888922 0.914378 1 1 1 1
  arc A309 (-26.5229, 44.3796) -> (-26.5992, 43.2637) centre (0.0409, 42.0024) ccw
  spline S105 degree 3 poles (-26.5678, 40.1949) (-26.3886, 40.2848) (-26.1528, 40.3948) (-25.8608, 40.5155) (-25.7043, 40.5765) (-25.5567, 40.6304) (-25.4183, 40.6777) (-25.2893, 40.7187) (-25.1698, 40.7541) (-25.06, 40.784) (-24.9601, 40.809) (-24.8704, 40.8295) (-24.7908, 40.846) (-24.7215, 40.8588) (-24.6627, 40.8683) (-24.597, 40.8778) (-24.5381, 40.8833) (-24.4833, 40.8898) (-24.4467, 40.8947) (-24.4111, 40.9002) (-24.3764, 40.9063) (-24.3426, 40.9129) (-24.3096, 40.92) (-24.2774, 40.9278) (-24.246, 40.9362) (-24.2153, 40.9453) (-24.1851, 40.9551) (-24.1554, 40.9657) (-24.1262, 40.9773) (-24.0972, 40.99) (-24.0684, 41.004) (-24.0396, 41.0196) (-24.0107, 41.037) (-23.9816, 41.0568) (-23.9521, 41.0796) (-23.9223, 41.1061) (-23.8925, 41.1371) (-23.8631, 41.1737) (-23.8352, 41.2168) (-23.8105, 41.2671) (-23.791, 41.3245) (-23.7796, 41.3849) (-23.7746, 41.5302) (-23.7882, 41.758) (-23.7793, 41.9859) (-23.7872, 42.1311) (-23.7999, 42.1913) (-23.8205, 42.2482) (-23.8463, 42.298) (-23.8751, 42.3406) (-23.9052, 42.3766) (-23.9357, 42.407) (-23.966, 42.4328) (-23.9959, 42.455) (-24.0255, 42.4742) (-24.0547, 42.491) (-24.0838, 42.506) (-24.1129, 42.5194) (-24.1421, 42.5315) (-24.1716, 42.5425) (-24.2015, 42.5525) (-24.2318, 42.5617) (-24.2628, 42.5701) (-24.2944, 42.5779) (-24.3267, 42.585) (-24.3598, 42.5915) (-24.3938, 42.5974) (-24.4286, 42.6027) (-24.4643, 42.6075) (-24.501, 42.6117) (-24.5559, 42.617) (-24.6149, 42.6213) (-24.6808, 42.6295) (-24.7398, 42.6378) (-24.8093, 42.6492) (-24.8892, 42.664) (-24.9794, 42.6826) (-25.0797, 42.7056) (-25.1901, 42.7333) (-25.3103, 42.7661) (-25.4401, 42.8046) (-25.5795, 42.849) (-25.7281, 42.8999) (-25.8859, 42.9576) (-26.1803, 43.0723) (-26.4183, 43.1775) (-26.5992, 43.2637) knots 0 0 0 0 0.085622 0.111078 0.134991 0.157361 0.178189 0.197474 0.215216 0.231415 0.246072 0.259186 0.270757 0.280785 0.28927 0.296213 0.309142 0.314525 0.319779 0.32491 0.329923 0.334826 0.339627 0.344336 0.348964 0.353525 0.358035 0.362514 0.366985 0.371475 0.37602 0.380661 0.385447 0.39044 0.395711 0.401345 0.407436 0.41408 0.421363 0.429333 0.437971 0.447155 0.455484 0.5 0.544516 0.552845 0.562029 0.570667 0.578637 0.58592 0.592564 0.598655 0.604289 0.60956 0.614553 0.619339 0.62398 0.628525 0.633015 0.637486 0.641965 0.646475 0.651036 0.655664 0.660373 0.665174 0.670077 0.67509 0.680221 0.685475 0.690858 0.703787 0.71073 0.719215 0.729243 0.740814 0.753928 0.768585 0.784784 0.802526 0.821811 0.842639 0.865009 0.888922 0.914378 1 1 1 1
  arc A310 (-26.5678, 40.1949) -> (-26.4686, 39.0807) centre (0.0409, 42.0024) ccw
  spline S106 degree 3 poles (-25.9574, 36.0546) (-25.7945, 36.1714) (-25.5789, 36.317) (-25.3093, 36.4819) (-25.1643, 36.5666) (-25.0269, 36.6429) (-24.8976, 36.7113) (-24.7766, 36.772) (-24.6641, 36.8256) (-24.5604, 36.8724) (-24.4657, 36.9127) (-24.3802, 36.947) (-24.3041, 36.9757) (-24.2377, 36.9991) (-24.1811, 37.0178) (-24.1177, 37.0375) (-24.0604, 37.0521) (-24.0073, 37.067) (-23.972, 37.0777) (-23.9377, 37.0887) (-23.9043, 37.1001) (-23.872, 37.1119) (-23.8405, 37.1241) (-23.8099, 37.1368) (-23.7802, 37.15) (-23.7513, 37.1638) (-23.723, 37.1782) (-23.6954, 37.1934) (-23.6683, 37.2094) (-23.6417, 37.2265) (-23.6154, 37.2448) (-23.5894, 37.2646) (-23.5636, 37.2864) (-23.5379, 37.3105) (-23.5123, 37.3376) (-23.4871, 37.3684) (-23.4624, 37.4037) (-23.4392, 37.4445) (-23.4184, 37.4914) (-23.4018, 37.545) (-23.3916, 37.6047) (-23.3897, 37.6662) (-23.4075, 37.8105) (-23.4566, 38.0333) (-23.4834, 38.2598) (-23.514, 38.402) (-23.536, 38.4594) (-23.5652, 38.5124) (-23.5985, 38.5576) (-23.6335, 38.5951) (-23.6689, 38.626) (-23.7038, 38.6512) (-23.7377, 38.672) (-23.7708, 38.6892) (-23.803, 38.7035) (-23.8345, 38.7156) (-23.8656, 38.7258) (-23.8964, 38.7345) (-23.9272, 38.7419) (-23.958, 38.7481) (-23.9891, 38.7534) (-24.0205, 38.7577) (-24.0524, 38.7612) (-24.0848, 38.7639) (-24.1178, 38.7659) (-24.1516, 38.7671) (-24.186, 38.7676) (-24.2212, 38.7675) (-24.2573, 38.7666) (-24.2941, 38.765) (-24.3492, 38.7617) (-24.4081, 38.7567) (-24.4745, 38.7544) (-24.5341, 38.7534) (-24.6045, 38.7538) (-24.6857, 38.7559) (-24.7777, 38.7602) (-24.8804, 38.7672) (-24.9938, 38.7773) (-25.1176, 38.7909) (-25.2519, 38.8086) (-25.3965, 38.8307) (-25.5513, 38.8577) (-25.7161, 38.89) (-26.0249, 38.9573) (-26.2764, 39.0239) (-26.4686, 39.0807) knots 0 0 0 0 0.085622 0.111078 0.134991 0.157361 0.178189 0.197474 0.215216 0.231415 0.246072 0.259186 0.270757 0.280785 0.28927 0.296213 0.309142 0.314525 0.319779 0.32491 0.329923 0.334826 0.339627 0.344336 0.348964 0.353525 0.358035 0.362514 0.366985 0.371475 0.37602 0.380661 0.385447 0.39044 0.395711 0.401345 0.407436 0.41408 0.421363 0.429333 0.437971 0.447155 0.455484 0.5 0.544516 0.552845 0.562029 0.570667 0.578637 0.58592 0.592564 0.598655 0.604289 0.60956 0.614553 0.619339 0.62398 0.628525 0.633015 0.637486 0.641965 0.646475 0.651036 0.655664 0.660373 0.665174 0.670077 0.67509 0.680221 0.685475 0.690858 0.703787 0.71073 0.719215 0.729243 0.740814 0.753928 0.768585 0.784784 0.802526 0.821811 0.842639 0.865009 0.888922 0.914378 1 1 1 1
  arc A311 (-25.9574, 36.0546) -> (-25.6852, 34.9697) centre (0.0409, 42.0024) ccw
  spline S107 degree 3 poles (-24.7069, 32.0608) (-24.5643, 32.2017) (-24.3741, 32.3791) (-24.1336, 32.5842) (-24.0036, 32.6905) (-23.8799, 32.7874) (-23.7629, 32.8752) (-23.6528, 32.9541) (-23.5501, 33.0246) (-23.455, 33.087) (-23.3677, 33.1417) (-23.2887, 33.1889) (-23.2181, 33.2291) (-23.1562, 33.2627) (-23.1032, 33.29) (-23.0436, 33.3193) (-22.9893, 33.3428) (-22.9392, 33.3658) (-22.9059, 33.3818) (-22.8738, 33.3981) (-22.8426, 33.4146) (-22.8125, 33.4313) (-22.7834, 33.4483) (-22.7552, 33.4656) (-22.7279, 33.4833) (-22.7014, 33.5015) (-22.6758, 33.5201) (-22.6508, 33.5394) (-22.6266, 33.5595) (-22.603, 33.5805) (-22.5799, 33.6027) (-22.5573, 33.6264) (-22.5352, 33.6519) (-22.5136, 33.6798) (-22.4926, 33.7105) (-22.4725, 33.7449) (-22.4537, 33.7836) (-22.4371, 33.8275) (-22.4239, 33.8771) (-22.4159, 33.9326) (-22.4151, 33.9932) (-22.4229, 34.0542) (-22.4631, 34.1939) (-22.5464, 34.4063) (-22.6084, 34.6259) (-22.6608, 34.7615) (-22.6914, 34.8148) (-22.7286, 34.8626) (-22.7685, 34.902) (-22.809, 34.9336) (-22.8488, 34.9585) (-22.8872, 34.978) (-22.924, 34.9932) (-22.9593, 35.005) (-22.9933, 35.0142) (-23.0264, 35.0212) (-23.0587, 35.0264) (-23.0905, 35.0301) (-23.122, 35.0326) (-23.1534, 35.0339) (-23.185, 35.0343) (-23.2167, 35.0336) (-23.2487, 35.0321) (-23.2812, 35.0297) (-23.3141, 35.0265) (-23.3476, 35.0224) (-23.3817, 35.0175) (-23.4165, 35.0118) (-23.4519, 35.0053) (-23.4881, 34.998) (-23.542, 34.9861) (-23.5994, 34.972) (-23.6646, 34.9593) (-23.7233, 34.9491) (-23.7929, 34.9384) (-23.8735, 34.9278) (-23.965, 34.9177) (-24.0675, 34.9085) (-24.181, 34.9007) (-24.3055, 34.8948) (-24.4409, 34.8913) (-24.5872, 34.8905) (-24.7443, 34.8929) (-24.9121, 34.899) (-25.2276, 34.9172) (-25.4864, 34.9436) (-25.6852, 34.9697) knots 0 0 0 0 0.085622 0.111078 0.134991 0.157361 0.178189 0.197474 0.215216 0.231415 0.246072 0.259186 0.270757 0.280785 0.28927 0.296213 0.309142 0.314525 0.319779 0.32491 0.329923 0.334826 0.339627 0.344336 0.348964 0.353525 0.358035 0.362514 0.366985 0.371475 0.37602 0.380661 0.385447 0.39044 0.395711 0.401345 0.407436 0.41408 0.421363 0.429333 0.437971 0.447155 0.455484 0.5 0.544516 0.552845 0.562029 0.570667 0.578637 0.58592 0.592564 0.598655 0.604289 0.60956 0.614553 0.619339 0.62398 0.628525 0.633015 0.637486 0.641965 0.646475 0.651036 0.655664 0.660373 0.665174 0.670077 0.67509 0.680221 0.685475 0.690858 0.703787 0.71073 0.719215 0.729243 0.740814 0.753928 0.768585 0.784784 0.802526 0.821811 0.842639 0.865009 0.888922 0.914378 1 1 1 1
  arc A312 (-24.7069, 32.0608) -> (-24.2683, 31.0318) centre (0.0409, 42.0024) ccw
  spline S108 degree 3 poles (-22.847, 28.3118) (-22.7282, 28.4732) (-22.5681, 28.6783) (-22.3627, 28.9185) (-22.2509, 29.0438) (-22.1439, 29.1588) (-22.042, 29.2638) (-21.9457, 29.359) (-21.8552, 29.4447) (-21.771, 29.5212) (-21.6934, 29.5888) (-21.6227, 29.6479) (-21.5593, 29.6987) (-21.5034, 29.7415) (-21.4553, 29.7767) (-21.4011, 29.815) (-21.3511, 29.8467) (-21.3052, 29.8773) (-21.2749, 29.8983) (-21.2456, 29.9194) (-21.2175, 29.9405) (-21.1903, 29.9617) (-21.1642, 29.9831) (-21.1391, 30.0046) (-21.1149, 30.0264) (-21.0916, 30.0484) (-21.0692, 30.0709) (-21.0476, 30.0938) (-21.0268, 30.1174) (-21.0067, 30.1419) (-20.9874, 30.1674) (-20.9688, 30.1944) (-20.951, 30.223) (-20.934, 30.2539) (-20.9181, 30.2876) (-20.9036, 30.3247) (-20.8911, 30.3659) (-20.8815, 30.4118) (-20.8762, 30.4629) (-20.877, 30.519) (-20.8857, 30.5789) (-20.9029, 30.6379) (-20.9645, 30.7697) (-21.08, 30.9664) (-21.1756, 31.1736) (-21.2485, 31.2993) (-21.2872, 31.3472) (-21.3314, 31.3886) (-21.377, 31.4212) (-21.4219, 31.4461) (-21.4651, 31.4645) (-21.506, 31.4777) (-21.5448, 31.487) (-21.5815, 31.4931) (-21.6166, 31.4968) (-21.6503, 31.4986) (-21.683, 31.4987) (-21.715, 31.4974) (-21.7465, 31.4949) (-21.7778, 31.4913) (-21.809, 31.4867) (-21.8402, 31.4811) (-21.8716, 31.4746) (-21.9033, 31.4672) (-21.9353, 31.4588) (-21.9677, 31.4496) (-22.0007, 31.4394) (-22.0341, 31.4284) (-22.0681, 31.4164) (-22.1027, 31.4035) (-22.154, 31.3833) (-22.2085, 31.3604) (-22.2709, 31.3377) (-22.3273, 31.3184) (-22.3944, 31.297) (-22.4723, 31.2739) (-22.5611, 31.2495) (-22.661, 31.2244) (-22.7719, 31.199) (-22.8939, 31.1737) (-23.027, 31.149) (-23.1714, 31.1253) (-23.3269, 31.1032) (-23.4937, 31.083) (-23.8081, 31.0515) (-24.0679, 31.0372) (-24.2683, 31.0318) knots 0 0 0 0 0.085622 0.111078 0.134991 0.157361 0.178189 0.197474 0.215216 0.231415 0.246072 0.259186 0.270757 0.280785 0.28927 0.296213 0.309142 0.314525 0.319779 0.32491 0.329923 0.334826 0.339627 0.344336 0.348964 0.353525 0.358035 0.362514 0.366985 0.371475 0.37602 0.380661 0.385447 0.39044 0.395711 0.401345 0.407436 0.41408 0.421363 0.429333 0.437971 0.447155 0.455484 0.5 0.544516 0.552845 0.562029 0.570667 0.578637 0.58592 0.592564 0.598655 0.604289 0.60956 0.614553 0.619339 0.62398 0.628525 0.633015 0.637486 0.641965 0.646475 0.651036 0.655664 0.660373 0.665174 0.670077 0.67509 0.680221 0.685475 0.690858 0.703787 0.71073 0.719215 0.729243 0.740814 0.753928 0.768585 0.784784 0.802526 0.821811 0.842639 0.865009 0.888922 0.914378 1 1 1 1
  arc A313 (-22.847, 28.3118) -> (-22.2528, 27.3641) centre (0.0409, 42.0024) ccw